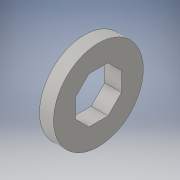
# Autodesk Inventor part: 40_Adapter_Lens_Phone
Saved by Autodesk Inventor 2016 (Build 200138000, 138)
## iProperties
Created: 2016-10-19
Part Number: 40_Adapter_Lens_Phone
Material: Generisch
Document SubType Name: Modeling
Designer: Bene
Density: 1 g/cm^3
Appearance: Vorgabe
Author: Bene
Autodesk Inventor part; units mm, degrees
ref_plane "YZ Plane" through (0, 0, 0) normal (1, 0, 0) x (0, 1, 0)
ref_plane "XZ Plane" through (0, 0, 0) normal (0, 1, 0) x (-1, 0, 0)
ref_plane "XY Plane" through (0, 0, 0) normal (0, 0, 1) x (1, 0, 0)
sketch "Skizze1" plane through (0, 0, 0) normal (1, 0, 0) x (0, 1, 0)
  circle A0 centre (0, 0) radius 4
  circle A1 centre (0, 0) radius 8
  line L0 (-4.1042, 1.688) -> (-1.7085, 4.0957)
  line L1 (-1.7085, 4.0957) -> (1.688, 4.1042)
  line L2 (1.688, 4.1042) -> (4.0957, 1.7085)
  line L3 (4.0957, 1.7085) -> (4.1042, -1.688)
  line L4 (4.1042, -1.688) -> (1.7085, -4.0957)
  line L5 (1.7085, -4.0957) -> (-1.688, -4.1042)
  line L6 (-1.688, -4.1042) -> (-4.0957, -1.7085)
  line L7 (-4.0957, -1.7085) -> (-4.1042, 1.688)
  dimension "d0" = 8
  dimension "d1" = 4
  dimension "d16" = 8.2
  constraints: 16 end point, 2 centre point, 2 coincident, 17 other
  measures "d0" diameter of A0
  measures "d1" radial gap between concentric circles of A0 A1
  measures "d16" distance between parallel lines of L4 L0
extrude "Extrusion1" add sketch "Skizze1" along normal blind 2.5 contours A1
sketch "Skizze6" plane through (0, 0, 0) normal (-1, 0, 0) x (0, 0, 1)
  circle A0 centre (0, 0) radius 8 projected
  circle A1 centre (0, 0) radius 6.25
  line L0 (4.1042, 1.688) -> (4.0957, -1.7085) projected
  line L1 (4.0957, -1.7085) -> (1.688, -4.1042) projected
  line L2 (1.688, -4.1042) -> (-1.7085, -4.0957) projected
  line L3 (-1.7085, -4.0957) -> (-4.1042, -1.688) projected
  line L4 (-4.1042, -1.688) -> (-4.0957, 1.7085) projected
  line L5 (-4.0957, 1.7085) -> (-1.688, 4.1042) projected
  line L6 (-1.688, 4.1042) -> (1.7085, 4.0957) projected
  line L7 (1.7085, 4.0957) -> (4.1042, 1.688) projected
  circle A2 centre (0, 0) radius 8 projected
  dimension "d13" = 12.5
  constraints: 1 centre point, 1 coincident
  measures "d13" diameter of A1
extrude "Extrusion3" add sketch "Skizze6" along normal blind 0.5 contours A1
